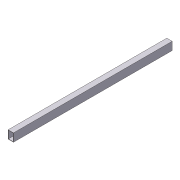
# Autodesk Inventor part: GE-12019-05
Saved by Autodesk Inventor 2012 (Build 160160000, 160)
## iProperties
Created: 2011-06-10
Part Number: GE-12019-05
Document SubType Name: Modeling
Designer: dfoster
Density: 2.71 g/cm^3
Material: Aluminum-6061
Mass: 3515.46 g
Surface Area: 8186.25 cm^2
Volume: 1297.22 cm^3
Description: Support, Inside
Title: Support, Inside
Author: dfoster
Autodesk Inventor part; units mm, degrees
ref_plane "YZ Plane" through (0, 0, 0) normal (1, 0, 0) x (0, 1, 0)
ref_plane "XZ Plane" through (0, 0, 0) normal (0, 1, 0) x (-1, 0, 0)
ref_plane "XY Plane" through (0, 0, 0) normal (0, 0, 1) x (1, 0, 0)
sketch "Sketch1" plane through (0, 0, 0) normal (0, 0, 1) x (1, 0, 0)
  line L0 (0, 0) -> (50.8, 0)
  line L1 (50.8, 0) -> (50.8, 76.2)
  line L2 (50.8, 76.2) -> (0, 76.2)
  line L3 (0, 76.2) -> (0, 0)
  line L4 (3.175, 73.025) -> (47.625, 73.025)
  line L5 (47.625, 73.025) -> (47.625, 3.175)
  line L6 (47.625, 3.175) -> (3.175, 3.175)
  line L7 (3.175, 3.175) -> (3.175, 73.025)
  dimension "d13" = 3.175
  dimension "d14" = 50.8
  dimension "d15" = 76.2
  dimension "d16" = 3.175
  dimension "d17" = 3.175
  dimension "d18" = 3.175
  constraints: 16 end point, 4 parallel, 2 perpendicular, 1 horizontal
  measures "d13" distance between parallel lines of L4 L2
  measures "d14" distance between parallel lines of L1 L3
  measures "d15" distance between parallel lines of L0 L2
  measures "d16" distance between parallel lines of L7 L3
  measures "d17" distance between parallel lines of L6 L0
  measures "d18" distance between parallel lines of L5 L1
extrude "Extrusion1" add sketch "Sketch1" along normal blind 1498.6
body "Solid1"
